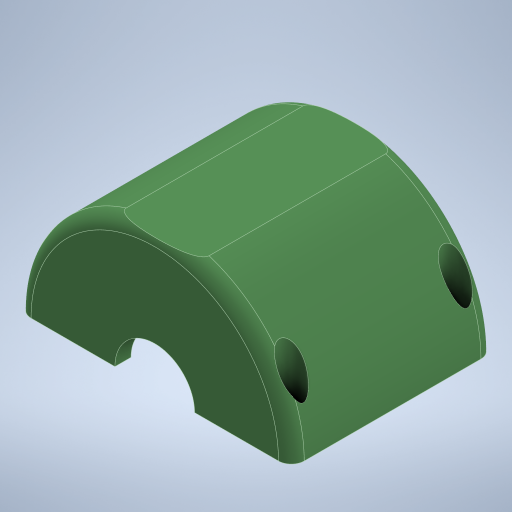
# Autodesk Inventor part: Base_1Up
Saved by Autodesk Inventor 2023 (Build 270158000, 158)
## iProperties
Created: 2024-07-31
Part Number: Base_1Up
Material: Generic
Document SubType Name: Modeling
Designer: Swoby
Density: 1 g/cm^3
Appearance: Default
Author: Swoby
Autodesk Inventor part; units mm, degrees
ref_plane "YZ Plane" through (0, 0, 0) normal (1, 0, 0) x (0, 1, 0)
ref_plane "XZ Plane" through (0, 0, 0) normal (0, 1, 0) x (-1, 0, 0)
ref_plane "XY Plane" through (0, 0, 0) normal (0, 0, 1) x (1, 0, 0)
sketch "Sketch1" plane through (0, 0, 0) normal (0, 0, 1) x (1, 0, 0)
  arc A0 (42.5, 0) -> (-42.5, 0) centre (0, 0) ccw
  line L0 (-42.5, 0) -> (42.5, 0)
  arc A1 (-42.5, 0) -> (42.5, 0) centre (0, 0) ccw construction
  dimension "d0" = 85
  constraints: 4 point on circle, 2 centre point, 2 end point, 1 coincident, 1 horizontal, 1 midpoint
  measures "d0" diameter of A0
extrude "Extrusion1" add sketch "Sketch1" along normal blind 63
fillet "Fillet1" radius 4 2 edges at (0, 42.5, 63) (0, 42.5, 0)
sketch "Sketch2" plane through (-38.5, 0, 0) normal (0, -1, 0) x (1, 0, 0)
  line L0 (38.5, 0) -> (38.5, 17.5847)
  line L1 (33.5, 1.6) -> (43.5, 1.6)
  line L2 (43.5, 1.6) -> (43.5, 0)
  line L3 (43.5, 0) -> (33.5, 0)
  line L4 (33.5, 0) -> (33.5, 1.6)
  line L5 (45.9, 3.1) -> (31.1, 3.1)
  line L6 (31.1, 3.1) -> (31.1, 1.6)
  line L7 (31.1, 1.6) -> (45.9, 1.6)
  line L8 (45.9, 1.6) -> (45.9, 3.1)
  line L9 (0, 0) -> (77, 0) projected
  line L10 (69.45, 43.7) -> (27.85, 43.7)
  line L11 (27.85, 3.1) -> (69.45, 3.1)
  line L12 (69.45, 10.6) -> (76.55, 10.6)
  line L13 (76.55, 10.6) -> (76.55, 14.3)
  line L14 (76.55, 14.3) -> (69.45, 14.3)
  line L15 (27.85, 14.3) -> (20.75, 14.3)
  line L16 (20.75, 14.3) -> (20.75, 10.6)
  line L17 (20.75, 10.6) -> (27.85, 10.6)
  line L18 (69.45, 3.1) -> (69.45, 10.6)
  line L19 (69.45, 14.3) -> (69.45, 34.4)
  line L20 (69.45, 39.8) -> (69.45, 43.7)
  line L21 (27.85, 10.6) -> (27.85, 3.1)
  line L22 (38.5, 63) -> (50.9, 63)
  line L23 (50.9, 63) -> (50.9, 53)
  line L24 (50.9, 53) -> (38.5, 53)
  line L25 (38.5, 53) -> (38.5, 63)
  line L26 (0, 63) -> (77, 63) projected
  line L27 (69.45, 39.8) -> (69.45, 34.4)
  line L28 (27.85, 39.8) -> (21.85, 39.8)
  line L29 (21.85, 39.8) -> (21.85, 34.4)
  line L30 (21.85, 34.4) -> (27.85, 34.4)
  line L31 (27.85, 43.7) -> (27.85, 39.8)
  line L32 (27.85, 34.4) -> (27.85, 14.3)
  point P0 (38.5, 1.6)
  point P1 (31.1, 2.35)
  point P2 (38.5, 3.1)
  point P3 (38.5, 3.1)
  dimension "d4" = 10
  dimension "d5" = 1.6
  dimension "d6" = 1.5
  dimension "d7" = 14.8
  dimension "d11" = 41.6
  dimension "d12" = 40.6
  dimension "d13" = 3.7
  dimension "d14" = 7.5
  dimension "d15" = 7.1
  dimension "d16" = 7.1
  dimension "d24" = 24.8
  dimension "d25" = 10
  dimension "d54" = 10.65
  dimension "d55" = 3.9
  dimension "d56" = 6
  dimension "d57" = 5.4
  constraints: 62 end point, 19 parallel, 11 perpendicular, 9 midpoint, 7 horizontal, 6 point on line, 4 collinear, 2 vertical
  measures "d4" distance of L2.end L3.end
  measures "d5" distance of L1.end L2.end
  measures "d6" distance of L7.end L5.start
  measures "d7" distance from line of point (31.1, 2.35) L8
  measures "d11" distance of L11.start L11.end
  measures "d12" distance between parallel lines of L11 L10
  measures "d13" distance of L12.end L13.end
  measures "d14" distance of L11.end L12.start
  measures "d15" distance of L12.start L12.end
  measures "d16" distance of L16.end L17.end
  measures "d24" diameter of L23 L0
  measures "d25" distance of L22.end L23.end
  measures "d54" distance from line of L21 point (38.5, 3.1)
  measures "d55" distance of L10.end L28.start
  measures "d56" distance of L29.end L30.end
  measures "d57" distance of L28.end L29.end
extrude "Extrusion2" cut sketch "Sketch2" against normal blind 10.6 contours L5 L11 L21 L17 L16 L15 L32 L30 L29 L28 L31 L10 L20 L27 L19 L14 L13 L12 L18
revolve "Revolution1" cut sketch "Sketch2" angle 360 about axis through (0, 0, 0) along (0, 0, 1) contours L0 L1 L2 L3 | L0 L5 L8 L7 L1 | L22 L23 L24 L25
sketch "Sketch3" plane through (42.5, 0, 4) normal (0, -1, 0) x (1, 0, 0)
  line L0 (-37.5, -2.4) -> (-37.5, -4) projected
  line L1 (-37.5, -4) -> (-4, -4) projected
  arc A0 (-4, -4) -> (0, 0) centre (-4, 0) ccw projected
  line L2 (0, 0) -> (0, 55) projected
  arc A1 (0, 55) -> (-4, 59) centre (-4, 55) ccw projected
  line L3 (-30.1, 59) -> (-4, 59) projected
  line L4 (-30.1, 59) -> (-30.1, 49) projected
  line L5 (-30.1, 49) -> (-54.9, 49) projected
  line L6 (-54.9, 49) -> (-54.9, 59) projected
  line L7 (-81, 59) -> (-54.9, 59) projected
  arc A2 (-81, 59) -> (-85, 55) centre (-81, 55) ccw projected
  line L8 (-85, 0) -> (-85, 55) projected
  arc A3 (-85, 0) -> (-81, -4) centre (-81, 0) ccw projected
  line L9 (-81, -4) -> (-47.5, -4) projected
  line L10 (-47.5, -4) -> (-47.5, -2.4) projected
  line L11 (-47.5, -2.4) -> (-49.9, -2.4) projected
  line L12 (-49.9, -2.4) -> (-49.9, -0.9) projected
  line L13 (-53.15, -0.9) -> (-53.15, 6.6) projected
  line L14 (-53.15, 6.6) -> (-60.25, 6.6) projected
  line L15 (-60.25, 6.6) -> (-60.25, 10.3) projected
  line L16 (-60.25, 10.3) -> (-53.15, 10.3) projected
  line L17 (-53.15, 35.8) -> (-53.15, 39.7) projected
  line L18 (-53.15, 39.7) -> (-11.55, 39.7) projected
  line L19 (-11.55, 39.7) -> (-11.55, 10.3) projected
  line L20 (-11.55, 10.3) -> (-4.45, 10.3) projected
  line L21 (-4.45, 10.3) -> (-4.45, 6.6) projected
  line L22 (-4.45, 6.6) -> (-11.55, 6.6) projected
  line L23 (-11.55, 6.6) -> (-11.55, -0.9) projected
  line L24 (-35.1, -0.9) -> (-35.1, -2.4) projected
  line L25 (-35.1, -2.4) -> (-37.5, -2.4) projected
  line L26 (-49.9, -0.9) -> (-53.15, -0.9) projected
  line L27 (-53.15, 10.3) -> (-53.15, 30.4) projected
  line L28 (-53.15, 30.4) -> (-59.15, 30.4) projected
  line L29 (-59.15, 30.4) -> (-59.15, 35.8) projected
  line L30 (-59.15, 35.8) -> (-53.15, 35.8) projected
  line L31 (-11.55, -0.9) -> (-35.1, -0.9) projected
  line L32 (-30.1, 49) -> (-42.5, 44.7)
  line L33 (-42.5, 44.7) -> (-62.15, 44.7)
  line L34 (-62.15, 44.7) -> (-62.15, 35.8)
  line L35 (-62.15, 35.8) -> (-59.15, 35.8)
  line L36 (-59.15, 30.4) -> (-72.15, 30.4)
  line L37 (-72.15, 30.4) -> (-72.15, 54)
  line L38 (-72.15, 54) -> (-54.9, 54)
  line L39 (-42.5, 49) -> (-42.5, 44.7)
  line L40 (-54.9, 54) -> (-42.5, 54)
  line L41 (-42.5, 54) -> (-42.5, 49)
  line L42 (-42.5, 49) -> (-54.9, 49)
  line L43 (-54.9, 49) -> (-54.9, 54)
  point P0 (-42.5, -4)
  point P1 (-72.15, 42.2)
  dimension "d59" = 5
  dimension "d60" = 5
  dimension "d61" = 12.85
  dimension "d62" = 10
  constraints: 24 end point, 4 perpendicular, 3 horizontal, 3 midpoint, 3 parallel, 1 vertical
  measures "d59" distance between parallel lines of L18 L33
  measures "d60" distance between parallel lines of L7 L38
  measures "d61" distance between parallel lines of L8 L37
  measures "d62" distance from line of point (-72.15, 42.2) L34
extrude "Extrusion3" cut sketch "Sketch3" against normal up to surface (10.6 mm away) contours L32 L39 L5 | L39 L33 L34 L35 L29 L36 L37 L38 L6 L5 | L5 L6 L40 L41
sketch "Sketch4" plane through (42.5, 0, 4) normal (0, -1, 0) x (1, 0, 0)
  line L0 (-11.55, 39.7) -> (-11.55, 10.3) projected
  line L1 (-11.55, 10.3) -> (-4.45, 10.3) projected
  line L2 (-4.45, 10.3) -> (-4.45, 6.6) projected
  line L3 (-4.45, 6.6) -> (-11.55, 6.6) projected
  line L4 (-11.55, 6.6) -> (-11.55, -0.9) projected
  line L5 (-35.1, -0.9) -> (-35.1, -2.4) projected
  line L6 (-35.1, -2.4) -> (-37.5, -2.4) projected
  line L7 (-37.5, -2.4) -> (-37.5, -4) projected
  line L8 (-37.5, -4) -> (-4, -4) projected
  arc A0 (-4, -4) -> (0, 0) centre (-4, 0) ccw projected
  line L9 (0, 0) -> (0, 55) projected
  arc A1 (0, 55) -> (-4, 59) centre (-4, 55) ccw projected
  line L10 (-30.1, 59) -> (-4, 59) projected
  line L11 (-30.1, 59) -> (-30.1, 49) projected
  line L12 (-42.5, 44.7) -> (-54.9, 49) projected
  line L13 (-54.9, 49) -> (-54.9, 59) projected
  line L14 (-81, 59) -> (-54.9, 59) projected
  arc A2 (-81, 59) -> (-85, 55) centre (-81, 55) ccw projected
  line L15 (-85, 0) -> (-85, 55) projected
  arc A3 (-85, 0) -> (-81, -4) centre (-81, 0) ccw projected
  line L16 (-81, -4) -> (-47.5, -4) projected
  line L17 (-47.5, -4) -> (-47.5, -2.4) projected
  line L18 (-47.5, -2.4) -> (-49.9, -2.4) projected
  line L19 (-49.9, -2.4) -> (-49.9, -0.9) projected
  line L20 (-53.15, -0.9) -> (-53.15, 6.6) projected
  line L21 (-53.15, 6.6) -> (-60.25, 6.6) projected
  line L22 (-60.25, 6.6) -> (-60.25, 10.3) projected
  line L23 (-60.25, 10.3) -> (-53.15, 10.3) projected
  line L24 (-53.15, 35.8) -> (-53.15, 39.7) projected
  line L25 (-53.15, 39.7) -> (-11.55, 39.7) projected
  circle A4 centre (-6, 53) radius 2
  circle A5 centre (-6, 2) radius 2
  circle A6 centre (-79, 53) radius 2
  circle A7 centre (-79.6196, 2) radius 2
  line L26 (-42.5, 49) -> (-42.5, 44.7) projected
  line L27 (-49.9, -0.9) -> (-53.15, -0.9) projected
  line L28 (-53.15, 10.3) -> (-53.15, 30.4) projected
  line L29 (-53.15, 30.4) -> (-59.15, 30.4) projected
  line L30 (-59.15, 30.4) -> (-59.15, 35.8) projected
  line L31 (-59.15, 35.8) -> (-53.15, 35.8) projected
  line L32 (-11.55, 39.7) -> (-11.55, 10.3) projected
  line L33 (-11.55, 10.3) -> (-4.45, 10.3) projected
  line L34 (-4.45, 10.3) -> (-4.45, 6.6) projected
  line L35 (-4.45, 6.6) -> (-11.55, 6.6) projected
  line L36 (-11.55, 6.6) -> (-11.55, -0.9) projected
  line L37 (-11.55, -0.9) -> (-35.1, -0.9) projected
  line L38 (-35.1, -0.9) -> (-35.1, -2.4) projected
  line L39 (-35.1, -2.4) -> (-37.5, -2.4) projected
  line L40 (-37.5, -2.4) -> (-37.5, -4) projected
  line L41 (-37.5, -4) -> (-4, -4) projected
  arc A8 (-4, -4) -> (0, 0) centre (-4, 0) ccw projected
  line L42 (0, 0) -> (0, 55) projected
  arc A9 (0, 55) -> (-4, 59) centre (-4, 55) ccw projected
  line L43 (-30.1, 59) -> (-4, 59) projected
  line L44 (-30.1, 59) -> (-30.1, 49) projected
  line L45 (-30.1, 49) -> (-42.5, 49) projected
  line L46 (-42.5, 49) -> (-42.5, 44.7) projected
  line L47 (-42.5, 44.7) -> (-54.9, 49) projected
  line L48 (-54.9, 49) -> (-54.9, 59) projected
  line L49 (-81, 59) -> (-54.9, 59) projected
  arc A10 (-81, 59) -> (-85, 55) centre (-81, 55) ccw projected
  line L50 (-85, 0) -> (-85, 55) projected
  arc A11 (-85, 0) -> (-81, -4) centre (-81, 0) ccw projected
  line L51 (-81, -4) -> (-47.5, -4) projected
  line L52 (-47.5, -4) -> (-47.5, -2.4) projected
  line L53 (-47.5, -2.4) -> (-49.9, -2.4) projected
  line L54 (-49.9, -2.4) -> (-49.9, -0.9) projected
  line L55 (-49.9, -0.9) -> (-53.15, -0.9) projected
  line L56 (-53.15, -0.9) -> (-53.15, 6.6) projected
  line L57 (-53.15, 6.6) -> (-60.25, 6.6) projected
  line L58 (-60.25, 6.6) -> (-60.25, 10.3) projected
  line L59 (-60.25, 10.3) -> (-53.15, 10.3) projected
  line L60 (-53.15, 10.3) -> (-53.15, 30.4) projected
  line L61 (-53.15, 30.4) -> (-59.15, 30.4) projected
  line L62 (-59.15, 30.4) -> (-59.15, 35.8) projected
  line L63 (-59.15, 35.8) -> (-53.15, 35.8) projected
  line L64 (-53.15, 35.8) -> (-53.15, 39.7) projected
  line L65 (-53.15, 39.7) -> (-11.55, 39.7) projected
  line L66 (-11.55, -0.9) -> (-35.1, -0.9) projected
  line L67 (-30.1, 49) -> (-42.5, 49) projected
  point P0 (-42.5, -4)
  dimension "d32" = 4
  dimension "d33" = 4
  dimension "d34" = 4
  dimension "d35" = 4
  dimension "d36" = 6
  dimension "d37" = 6
  dimension "d38" = 6
  dimension "d39" = 6
  dimension "d40" = 6
  dimension "d41" = 6
  dimension "d42" = 5.3804
  dimension "d43" = 6
  constraints: 4 centre point
  measures "d32" diameter of A4
  measures "d33" diameter of A5
  measures "d34" diameter of A6
  measures "d35" diameter of A7
  measures "d36" distance from line of L15 A6.centre
  measures "d37" distance from line of L14 A6.centre
  measures "d38" distance from line of A4.centre L9
  measures "d39" distance from line of L10 A4.centre
  measures "d40" distance from line of L9 A5.centre
  measures "d41" distance from line of L8 A5.centre
  measures "d42" distance from line of L15 A7.centre
  measures "d43" distance from line of L16 A7.centre
extrude "Extrusion4" cut sketch "Sketch4" against normal through all contours A4 | A5 | A6 | A7
ref_plane "Work Plane1" through (42.5, 6, 4) normal (0, -1, 0) x (1, 0, 0)
sketch "Sketch5" plane through (42.5, 6, 4) normal (0, -1, 0) x (1, 0, 0)
  circle A0 centre (-6, 53) radius 3.75
  circle A1 centre (-6, 2) radius 3.75
  circle A2 centre (-79.6196, 2) radius 3.75
  circle A3 centre (-79, 53) radius 3.75
  point P0 (-42.5, -4)
  dimension "d47" = 7.5
  dimension "d48" = 7.5
  dimension "d49" = 7.5
  dimension "d50" = 7.5
  constraints: 4 centre point, 8 other
  measures "d47" diameter of A0
  measures "d48" diameter of A1
  measures "d49" diameter of A2
  measures "d50" diameter of A3
extrude "Extrusion5" cut sketch "Sketch5" against normal through all
fillet "Fillet2" radius 4 2 edges at (-19.65, 5.3, 48.7) (-29.65, 5.3, 58)
sketch "Sketch6" plane through (0, 0, 0) normal (1, 0, 0) x (0, 1, 0)
  arc A0 (42.5, 59) -> (38.5, 63) centre (38.5, 59) ccw projected
  line L0 (42.5, 4) -> (42.5, 59) projected
  arc A1 (38.5, 0) -> (42.5, 4) centre (38.5, 4) ccw projected
  line L1 (40.5, 62.4641) -> (40.5, 0.5359)
  point P0 (0, 0)
  dimension "d64" = 2
  constraints: 2 end point, 2 point on circle, 1 vertical
  measures "d64" distance between parallel lines of L1 L0
extrude "Extrusion6" cut sketch "Sketch6" along normal through all both and the other way through all
body "Solid1"
